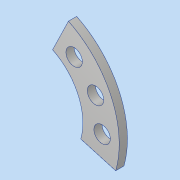
# Autodesk Inventor part: gearboxBearingHolderForward
Saved by Autodesk Inventor 2017.3 (Build 213256000, 256)
## iProperties
Created: 2018-09-02
Part Number: gearboxBearingHolderForward
Material: Aluminum 6061
Document SubType Name: Modeling
Designer: Derek Wider
Density: 2.7 g/cm^3
Appearance: Aluminum - Flat
Author: Derek Wider
Autodesk Inventor part; units mm, degrees
ref_plane "YZ Plane" through (0, 0, 0) normal (1, 0, 0) x (0, 1, 0)
ref_plane "XZ Plane" through (0, 0, 0) normal (0, 1, 0) x (-1, 0, 0)
ref_plane "XY Plane" through (0, 0, 0) normal (0, 0, 1) x (1, 0, 0)
sketch "Sketch2" plane through (0, 0, 0) normal (0, 0, 1) x (1, 0, 0)
  circle A0 centre (28.194, 0) radius 3.175
  circle A1 centre (25.645, 11.7147) radius 3.175
  circle A2 centre (17.397, 20.4153) radius 3.175
  line L0 (0, 0) -> (28.194, 0) construction
  line L1 (25.645, 11.7147) -> (0, 0) construction
  line L2 (17.397, 20.4153) -> (0, 0) construction
  line L3 (19.9596, -5.7253) -> (33.4491, -9.5947)
  line L4 (9.069, 18.6793) -> (15.1982, 31.3036)
  arc A3 (19.9596, -5.7253) -> (9.069, 18.6793) centre (0, 0) ccw
  arc A4 (33.4491, -9.5947) -> (15.1982, 31.3036) centre (0, 0) ccw
  dimension "d2" = 6.35
  dimension "d4" = 28.194
  dimension "d5" = 26.8224
  dimension "d6" = 11.9888
  dimension "d7" = 11.9888
  dimension "d9" = 41.529
  dimension "d11" = 69.596
  constraints: 10 end point, 5 centre point, 4 line through centre, 4 point on circle, 2 coincident, 2 equal radius, 1 equal length, 1 horizontal
  measures "d2" diameter of A0
  measures "d4" distance of L0.start L0.end
  measures "d5" distance of L2.start L0.start
  measures "d6" distance of L1.start L0.end
  measures "d7" distance of L1.start L2.start
  measures "d9" diameter of A3
  measures "d11" diameter of A4
extrude "Extrusion1" add sketch "Sketch2" along normal blind 3.175
body "Solid1"
